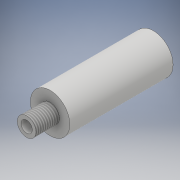
# Autodesk Inventor part: Lagertopf
Saved by Autodesk Inventor 2017 (Build 210142000, 142)
## iProperties
Created: 2019-06-21
Part Number: Lagertopf
Material: Generic
Document SubType Name: Modeling
Designer: Ole Simmering
Density: 1 g/cm^3
Appearance: Default
Author: Ole Simmering
Autodesk Inventor part; units mm, degrees
ref_plane "YZ Plane" through (0, 0, 0) normal (1, 0, 0) x (0, 1, 0)
ref_plane "XZ Plane" through (0, 0, 0) normal (0, 1, 0) x (-1, 0, 0)
ref_plane "XY Plane" through (0, 0, 0) normal (0, 0, 1) x (1, 0, 0)
sketch "Sketch1" plane through (0, 0, 0) normal (0, 0, 1) x (1, 0, 0)
  line L0 (0, 0) -> (0, -25) construction
  line L1 (6, 5) -> (6, -25)
  line L2 (6, -25) -> (10, -25)
  line L3 (10, -25) -> (10, 0)
  line L4 (0, 0) -> (6, 0) construction
  line L5 (10, 0) -> (21, 0)
  line L6 (21, 0) -> (21, 110)
  line L7 (6, 5) -> (16, 5)
  line L8 (16, 5) -> (16, 110)
  line L9 (21, 110) -> (16, 110)
  line L10 (0, 0) -> (0, 121) construction
  point P0 (3, 0)
  dimension "d0" = 12
  dimension "d1" = 20
  dimension "d2" = 25
  dimension "d6" = 110
  dimension "d8" = 5
  dimension "d9" = 5
  dimension "d11" = 32
  constraints: 22 end point, 3 horizontal, 3 perpendicular, 3 point on line, 3 vertical, 1 midpoint
  measures "d0" diameter of L1 L0
  measures "d1" diameter of L3 L0
  measures "d2" distance of L2.end L3.end
  measures "d6" distance of L5.end L6.end
  measures "d8" distance from line of L1.start L5
  measures "d9" distance between parallel lines of L6 L8
  measures "d11" diameter of L8 L10
revolve "Revolution1" add sketch "Sketch1" angle 360 about axis through (0, 0, 0) along (0, -1, 0)
thread "Thread1" size "M20x2.5" class "6g" standard "ANSI Metric M Profile" full length
thread "Thread3" size "M32x2" class "6H" standard "ANSI Metric M Profile" length 10
body "Solid1"
